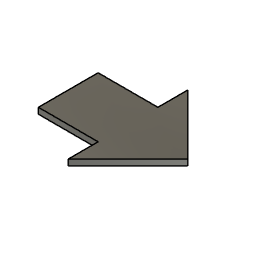
Arrow (Autodesk Fusion 360 design; units mm, degrees)
Autodesk Fusion 360 part; units mm, degrees
sketch "スケッチ1" plane through (0, 0, 0) normal (0, 0, 1) x (1, 0, 0)
  line L0 (0, 25) -> (50, 25)
  line L1 (50, -25) -> (0, -25)
  line L2 (0, -25) -> (0, 25)
  line L3 (50, 25) -> (50, 50)
  line L4 (50, 50) -> (100, 0)
  line L5 (100, 0) -> (50, -50)
  line L6 (50, -50) -> (50, -25)
  line L7 (0, 0) -> (100, 0) construction
  dimension "d2" = 100
  dimension "d3" = 50
  dimension "d4" = 50
  dimension "d5" = 100
  constraint horizontal L0
  constraint horizontal L1
  constraint vertical L2
  constraint perpendicular L0 L3
  constraint perpendicular L1 L6
  constraint equal L3 L6
  constraint collinear L3 L6
  constraint midpoint L7.start L2
  constraint coincident L7.start origin
  constraint horizontal L7
  measures "d2" distance of L7.start L4.end
  measures "d3" distance of L1.start L1.end
  measures "d4" vertical distance of L0.start L1.start
  measures "d5" distance of L3.end L5.end
extrude "押し出し1" add sketch "スケッチ1" along normal blind 5
